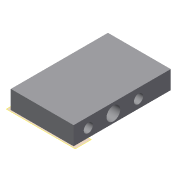
# Autodesk Inventor part: 01_Slide_camera_x_v0
Saved by Autodesk Inventor 2019.4 (Build 234330000, 330)
## iProperties
Created: 2020-10-27
Part Number: 01_Slide_camera_x_v0
Material: Generic
Document SubType Name: Modeling
Designer: diederichbenedict
Density: 1 g/cm^3
Appearance: Default
Author: diederichbenedict
Autodesk Inventor part; units mm, degrees
ref_plane "YZ Plane" through (0, 0, 0) normal (1, 0, 0) x (0, 1, 0)
ref_plane "XZ Plane" through (0, 0, 0) normal (0, 1, 0) x (-1, 0, 0)
ref_plane "XY Plane" through (0, 0, 0) normal (0, 0, 1) x (1, 0, 0)
ref_plane "Work Plane5" through (13.4046, 50.1721, 72.2727) normal (0, 1, 0) x (1, 0, 0)
sketch "Sketch7" plane through (13.4046, 50.1721, 72.2727) normal (0, 1, 0) x (1, 0, 0)
  circle A0 centre (6.5, 6.5) radius 2.5 construction
  circle A1 centre (48.5, 6.5) radius 2.5 construction
  line L0 (55, 2) -> (55, 11) construction
  line L1 (55, 35) -> (55, 44) construction
  circle A2 centre (48.5, 39.5) radius 2.5 construction
  circle A3 centre (6.5, 39.5) radius 2.5 construction
  line L2 (0, 35) -> (0, 44) construction
  line L3 (16.5, 85.8) -> (16.5, 84) construction
  line L4 (38.5, 85.8) -> (38.5, 84) construction
  line L5 (38.5, 84) -> (16.5, 84) construction
  line L6 (2, 0) -> (53, 0) construction
  line L7 (0, 0.7299) -> (55, 0.7299)
  line L8 (55, 0.7299) -> (55, 85.8)
  line L9 (55, 85.8) -> (0, 85.8)
  line L10 (0, 85.8) -> (0, 0.7299)
  point P0 (-13.4046, 72.2727)
  constraints: 22 end point, 5 vertical, 4 centre point, 3 horizontal, 2 parallel, 1 perpendicular, 1 point on line, 20 other
extrude "Extrusion7" add sketch "Sketch7" along normal blind 16
sketch "Sketch8" plane through (13.4046, 50.1721, -13.5273) normal (-1, 0, 0) x (0, 0, 1)
  circle A0 centre (50.2042, 7.5) radius 4
  circle A1 centre (72.2042, 7.5) radius 4
  circle A2 centre (28.2042, 7.5) radius 4
  circle A3 centre (50.2042, 7.5) radius 6
  point P0 (13.5273, -50.1721)
  dimension "d35" = 8
  dimension "d36" = 8
  dimension "d37" = 0
  dimension "d38" = 22
  dimension "d39" = 22
  dimension "d40" = 12
  constraints: 4 centre point, 1 coincident, 2 other
  measures "d35" diameter of A1
  measures "d36" diameter of A2
  measures "d37" vertical distance of A1.centre A0.centre
  measures "d38" distance of A0.centre A1.centre
  measures "d39" distance of A2.centre A0.centre
  measures "d40" diameter of A3
extrude "Extrusion8" cut sketch "Sketch8" against normal through all contours A0 | A1 | A2 | A3
sketch "Sketch9" plane through (13.4046, 50.1721, 72.2727) normal (0, -1, 0) x (1, 0, 0)
  circle A0 centre (6.5, -6.5) radius 2.5
  circle A1 centre (48.5, -6.5) radius 2.5
  circle A2 centre (48.5, -44.5) radius 2.5
  line L0 (4.5, -51) -> (4.5, 149)
  circle A3 centre (6.5, -44.5) radius 2.5
  point P0 (-13.4046, -72.2727)
  constraints: 4 centre point, 2 end point, 1 vertical, 10 other
hole "Hole1" at (19.9046, 50.1721, 65.7727) at (61.9046, 50.1721, 65.7727) at (61.9046, 50.1721, 27.7727) at (19.9046, 50.1721, 27.7727) direction (0, 1, 0) diameter 2.9 end through all
sketch "Sketch10" plane through (68.4046, 50.1721, -13.5273) normal (0, 0, -1) x (-1, 0, 0)
  circle A0 centre (39, -26) radius 1
  circle A1 centre (16, -26) radius 1
  circle A2 centre (16, -3) radius 1
  circle A3 centre (39, -3) radius 1.1
  circle A4 centre (27.5, -14.5) radius 12
  circle A5 centre (27.5, -14.5) radius 10.8
  line L0 (55, 0) -> (0, 0) projected
  line L1 (11.5, -29) -> (43.5, -29)
  line L2 (43.5, -29) -> (43.5, 0)
  line L3 (43.5, 0) -> (11.5, 0)
  line L4 (11.5, 0) -> (11.5, -29)
  line L5 (11.5, -29) -> (43.5, 0) construction
  line L6 (43.5, -29) -> (11.5, 0) construction
  line L7 (43.5, -29) -> (55, 0)
  line L8 (11.5, -29) -> (0, 0)
  line L9 (0, 0) -> (11.5, 0)
  line L10 (43.5, 0) -> (55, 0)
  point P0 (68.4046, -50.1721)
  dimension "d50" = 24
  dimension "d51" = 32
  constraints: 20 end point, 6 centre point, 2 collinear, 2 midpoint, 2 parallel, 1 horizontal, 1 perpendicular, 1 point on line, 10 other
  measures "d50" diameter of A4
  measures "d51" distance of L3.end L2.end
extrude "Extrusion9" add sketch "Sketch10" against normal blind 10 contours L7 L2 L0 | L2 L1 L4 L0 | L4 L8 L0
body "Solid2"
